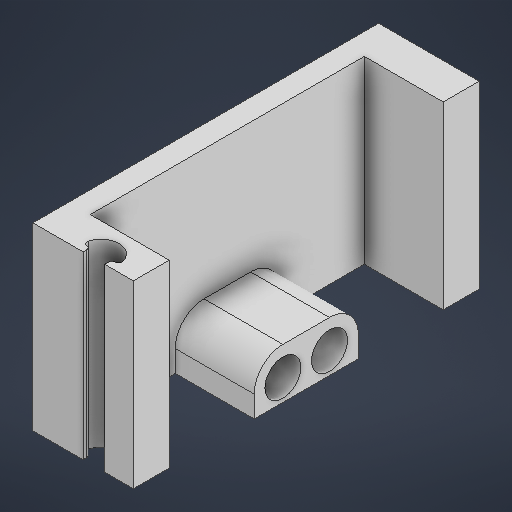
# Autodesk Inventor part: Pixy2 cover
Saved by Autodesk Inventor 2026 (Build 300175050, 175E)
## iProperties
Created: 2025-10-30
Part Number: Pixy2 cover
Material: Generic
Document SubType Name: Modeling
Designer: aduwa
Density: 1 g/cm^3
Appearance: Default
Author: aduwa
Autodesk Inventor part; units mm, degrees
ref_plane "YZ Plane" through (0, 0, 0) normal (1, 0, 0) x (0, 1, 0)
ref_plane "XZ Plane" through (0, 0, 0) normal (0, 1, 0) x (-1, 0, 0)
sketch "Sketch1" plane through (0, 0, 0) normal (1, 0, 0) x (0, 1, 0)
  line L0 (0, 0) -> (-25.1, 0)
  line L1 (-25.1, 0) -> (-25.1, -38.2)
  line L2 (-25.1, -38.2) -> (0, -38.2)
  line L3 (0, -38.2) -> (0, 0)
  circle A0 centre (-22.1, -15.85) radius 2.5
  circle A1 centre (-22.1, -22.35) radius 2.5
  arc A2 (-18.1, -15.85) -> (-25.1, -18.4958) centre (-22.1, -15.85) ccw
  arc A3 (-25.1, -19.7042) -> (-18.1, -22.35) centre (-22.1, -22.35) ccw
  line L4 (-18.1, -15.85) -> (-18.1, -22.35)
  line L5 (-22.1, -11.85) -> (-25.1, -11.85)
  line L6 (-22.1, -26.35) -> (-25.1, -26.35)
  line L7 (0, 0) -> (-25.1, 0)
  line L8 (-25.1, 0) -> (-25.1, 5)
  line L9 (-25.1, 5) -> (0, 5)
  line L10 (0, 5) -> (0, 0)
  line L11 (0, -38.2) -> (-25.1, -38.2)
  line L12 (-25.1, -38.2) -> (-25.1, -43.2)
  line L13 (-25.1, -43.2) -> (0, -43.2)
  line L14 (0, -43.2) -> (0, -38.2)
  point P0 (-25.1, -19.1)
  point P1 (-25.1, -13.2042)
  point P2 (-25.1, -24.9958)
  dimension "d0" = 38.2
  dimension "d1" = 25.1
  dimension "d2" = 5
  dimension "d3" = 6.5
  dimension "d4" = 3
  dimension "d5" = 3.25
  dimension "d6" = 8
  dimension "d11" = 5
  dimension "d12" = 5
  constraints: 30 end point, 6 parallel, 6 point on circle, 5 perpendicular, 5 point on line, 4 centre point, 3 horizontal, 3 tangent, 2 coincident, 2 equal radius, 1 midpoint, 1 vertical alignment
  measures "d0" distance of L1.end L0.end
  measures "d1" distance of L1.end L2.end
  measures "d2" diameter of A0
  measures "d3" distance of A1.centre A0.centre
  measures "d4" distance from line of L1 A1.centre
  measures "d5" vertical distance of point (-25.1, -19.1) A0.centre
  measures "d6" diameter of A2
  measures "d11" distance of L7.end L8.end
  measures "d12" distance of L12.end L11.end
extrude "Extrusion1" add sketch "Sketch1" against normal blind 3 contours L3 L2 L1 L6 A3 L4 A2 L5 L0 | L0 L8 L9 L10 | L14 L13 L12 L2 | L5 A2 L1 | A2 L4 A3 L1 | L1 A3 L6 | A0 | A1
extrude "Extrusion2" add sketch "Sketch1" along normal blind 11 contours L0 L8 L9 L10 | L14 L13 L12 L2 | L5 A2 L1 | A2 L4 A3 L1 | L1 A3 L6
sketch "Sketch2" plane through (-3, -25.1, 5) normal (0, 0, 1) x (1, 0, 0)
  circle A0 centre (7, 20.1) radius 2.6
  line L0 (0, 25.1) -> (14, 25.1) projected
  circle A1 centre (7, 8.1) radius 2.6
  point P0 (3, 25.1)
  point P1 (7, 25.1)
  dimension "d13" = 5.2
  dimension "d14" = 5
  dimension "d15" = 12
  constraints: 2 centre point, 1 equal radius, 1 midpoint, 1 vertical alignment
  measures "d13" diameter of A0
  measures "d14" distance from line of L0 A0.centre
  measures "d15" distance of A1.centre A0.centre
extrude "Extrusion3" [suppressed]
ref_plane "Work Plane1" through (-3, -25.1, -19.1) normal (0, 0, 1) x (1, 0, 0)
sketch "Sketch3" plane through (-3, 0, 5) normal (0, 1, 0) x (1, 0, 0)
  line L0 (14, 48.2) -> (0, 48.2) projected
  line L1 (0, 0) -> (0, 48.2) projected
  line L2 (0, 0) -> (14, 0) projected
  line L3 (14, 5) -> (14, 0) projected
  line L4 (3, 5) -> (14, 5) projected
  line L5 (3, 43.2) -> (3, 5) projected
  line L6 (3, 43.2) -> (14, 43.2) projected
  line L7 (14, 48.2) -> (14, 43.2) projected
  arc A0 (10.9206, 1.625) -> (6.0794, 1.625) centre (8.5, 1) ccw
  line L8 (10, 0.5) -> (10, 0)
  line L9 (7, 0.5) -> (7, 0)
  arc A1 (7, 0.5) -> (6.5, 1) centre (6.5, 0.5) ccw
  arc A2 (10.5, 1) -> (10, 0.5) centre (10.5, 0.5) ccw
  line L10 (6.5, 1) -> (6, 1)
  arc A3 (11, 1) -> (6, 1) centre (8.5, 1) ccw
  line L11 (10.5, 1) -> (11, 1)
  point P0 (8.5, 5)
  point P1 (7, 1)
  point P2 (10, 1)
  point P3 (10.9206, 1.625)
  point P4 (6.0794, 1.625)
  dimension "d23" = 5
  dimension "d26" = 1.5
  dimension "d28" = 1.5
  dimension "d31" = 0.5
  constraints: 10 point on circle, 8 end point, 4 centre point, 3 point on line, 2 horizontal, 2 midpoint, 2 perpendicular, 2 tangent, 1 coincident, 1 equal radius, 1 vertical alignment
  measures "d23" diameter of A0
  measures "d26" distance from line of L8 A0.centre
  measures "d28" distance from line of A0.centre L9
  measures "d31" radius of A1
extrude "Extrusion4" cut sketch "Sketch3" against normal through all contours L9 A1 L10 A3 A0 L11 A2 L8 L2
fillet "Fillet1" radius 0.5 2 edges at (3, -12.55, 4) (8, -12.55, 4)
body "Solid1"
